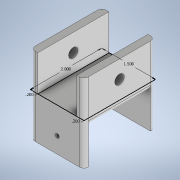
# Autodesk Inventor part: Sample Holder end for 8020-thruhole-widestance
Saved by Autodesk Inventor 2020 (Build 240168000, 168)
## iProperties
Created: 2022-02-15
Part Number: Sample Holder end for 8020-thruhole-widestance
Material: Generic
Document SubType Name: Modeling
Designer: Beaucage
Density: 1 g/cm^3
Appearance: Default
Author: Beaucage
Autodesk Inventor part; units mm, degrees
ref_plane "YZ Plane" through (0, 0, 0) normal (1, 0, 0) x (0, 1, 0)
ref_plane "XZ Plane" through (0, 0, 0) normal (0, 1, 0) x (-1, 0, 0)
ref_plane "XY Plane" through (0, 0, 0) normal (0, 0, 1) x (1, 0, 0)
sketch "Sketch1" plane through (0, 0, 0) normal (0, 1, 0) x (-1, 0, 0)
  line L0 (0, 0) -> (38.1, 0)
  line L1 (38.1, 0) -> (38.1, -50.8)
  line L2 (38.1, -50.8) -> (0, -50.8)
  line L3 (0, -50.8) -> (0, 0)
  line L4 (38.1, -50.8) -> (33.02, -50.8)
  line L5 (33.02, -50.8) -> (33.02, 0)
  line L6 (33.02, 0) -> (38.1, 0)
  line L7 (38.1, 0) -> (38.1, -50.8)
  line L8 (0, -50.8) -> (5.08, -50.8)
  line L9 (5.08, -50.8) -> (5.08, 0)
  line L10 (5.08, 0) -> (0, 0)
  line L11 (0, 0) -> (0, -50.8)
  dimension "d0" = 38.1
  dimension "d1" = 50.8
  dimension "d2" = 5.08
  dimension "d3" = 5.08
  constraints: 24 end point, 6 parallel, 3 horizontal, 3 perpendicular, 2 point on line
  measures "d0" distance of L1.end L2.end
  measures "d1" distance of L0.end L1.end
  measures "d2" distance of L5.end L6.end
  measures "d3" distance of L10.end L9.end
extrude "Extrusion1" add sketch "Sketch1" along normal blind 25.4 contours L0 L9 L2 L3 | L0 L1 L2 L5
extrude "Extrusion2" add sketch "Sketch1" against normal blind 5.08
sketch "Sketch2" plane through (0, 25.4, 0) normal (1, 0, 0) x (0, 0, -1)
  line L0 (50.8, 0) -> (0, 0) projected
  line L1 (25.4, 0) -> (25.4, -12.7)
  point P0 (0, -25.4)
  dimension "d8" = 12.7
  constraints: 2 end point, 1 midpoint, 1 vertical
  measures "d8" distance of L1.start L1.end
hole "Hole1" at (0, 12.7, -25.4) direction (-1, 0, 0) diameter 6.7564 end through all clearance for "Socket Head Cap Screw" size "1/4" standard "Ansi Unified Screw Threads"
sketch "Sketch3" plane through (0, -5.08, 0) normal (0, -1, 0) x (1, 0, 0)
  line L0 (0, -50.8) -> (-5.08, -50.8) projected
  line L1 (0, -50.8) -> (0, -38.1)
  line L2 (0, 0) -> (0, -50.8) projected
  line L3 (0, -38.1) -> (0, -12.7)
  line L4 (0, -38.1) -> (-19.05, -38.1)
  line L5 (0, -12.7) -> (-19.05, -12.7)
  line L6 (-38.1, -50.8) -> (-38.1, 0) projected
  line L7 (0, -39.6875) -> (-38.1, -39.6875)
  line L8 (-38.1, -39.6875) -> (-38.1, -36.5125)
  line L9 (-38.1, -36.5125) -> (0, -36.5125)
  line L10 (0, -36.5125) -> (0, -39.6875)
  line L11 (0, -39.6875) -> (-38.1, -36.5125) construction
  line L12 (-38.1, -39.6875) -> (0, -36.5125) construction
  line L13 (0, -11.1125) -> (-38.1, -11.1125)
  line L14 (-38.1, -11.1125) -> (-38.1, -14.2875)
  line L15 (-38.1, -14.2875) -> (0, -14.2875)
  line L16 (0, -14.2875) -> (0, -11.1125)
  line L17 (0, -11.1125) -> (-38.1, -14.2875) construction
  line L18 (-38.1, -11.1125) -> (0, -14.2875) construction
  line L19 (-38.1, 0) -> (-38.1, -50.8) projected
  line L20 (-38.1, 0) -> (0, 0)
  line L21 (0, 0) -> (0, -3.175)
  line L22 (0, -3.175) -> (-38.1, -3.175)
  line L23 (-38.1, -3.175) -> (-38.1, 0)
  line L24 (0, -50.8) -> (-38.1, -50.8)
  line L25 (-38.1, -50.8) -> (-38.1, -47.625)
  line L26 (-38.1, -47.625) -> (0, -47.625)
  line L27 (0, -47.625) -> (0, -50.8)
  dimension "d16" = 12.7
  dimension "d17" = 25.4
  dimension "d18" = 19.05
  dimension "d19" = 3.175
  dimension "d20" = 3.175
  dimension "d32" = 3.175
  dimension "d33" = 3.175
  constraints: 48 end point, 8 parallel, 6 horizontal, 5 point on line, 4 midpoint, 4 perpendicular, 2 other
  measures "d16" distance of L0.start L1.end
  measures "d17" distance of L1.end L3.end
  measures "d18" distance of L1.end L4.end
  measures "d19" distance of L7.end L8.end
  measures "d20" distance of L14.end L13.end
  measures "d32" distance of L20.end L21.end
  measures "d33" distance of L24.end L25.end
extrude "Extrusion3" add sketch "Sketch3" along normal blind 25.4 contours L0 L24 L6 L26 L1 | L6 L20 L2 L22
sketch "Sketch4" plane through (-38.1, -5.08, 0) normal (0, 0, 1) x (1, 0, 0)
  line L0 (38.1, -25.4) -> (19.05, -25.4)
  line L1 (19.05, -25.4) -> (19.05, -13.97)
  point P0 (38.1, 5.08)
  dimension "d23" = 11.43
  constraints: 4 end point, 1 vertical
  measures "d23" distance of L0.end L1.end
hole "Hole2" at (-19.05, -19.05, 0) direction (0, 0, -1) diameter 2.8575 end through all
fillet "Fillet1" radius 3.175 6 edges at (-38.1, -2.54, 0) (0, -2.54, 0) (0, -2.54, -50.8) (-38.1, -2.54, -50.8) (0, -5.08, -25.4) (-38.1, -5.08, -25.4)
body "Solid1"
